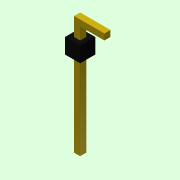
# Autodesk Inventor part: Pin-connector-angled
Saved by Autodesk Inventor 2015 (Build 190159000, 159)
## iProperties
Created: 2015-06-24
Part Number: Pin-connector-angled
Material: Generic
Document SubType Name: Modeling
Designer: Openlab
Density: 1 g/cm^3
Appearance: Default
Author: Openlab
Autodesk Inventor part; units mm, degrees
ref_plane "YZ Plane" through (0, 0, 0) normal (1, 0, 0) x (0, 1, 0)
ref_plane "XZ Plane" through (0, 0, 0) normal (0, 1, 0) x (-1, 0, 0)
ref_plane "XY Plane" through (0, 0, 0) normal (0, 0, 1) x (1, 0, 0)
sketch "Sketch1" plane through (0, 0, 0) normal (0, 1, 0) x (-1, 0, 0)
  line L0 (0, 0) -> (5, 0)
  line L1 (5, 0) -> (5, -19.5)
  line L2 (5, -19.5) -> (4, -19.5)
  line L3 (4, -19.5) -> (4, -1)
  line L4 (4, -1) -> (0, -1)
  line L5 (0, -1) -> (0, 0)
  line L6 (5.75, -3) -> (3.25, -3)
  line L7 (3.25, -3) -> (3.25, -5.5)
  line L8 (3.25, -5.5) -> (5.75, -5.5)
  line L9 (5.75, -5.5) -> (5.75, -3)
  line L10 (4.5, -1.8535) -> (4.5, -3.6396) construction
  dimension "d0" = 4
  dimension "d1" = 5
  dimension "d2" = 2.5
  dimension "d3" = 2.5
  dimension "d4" = 2
  dimension "d5" = 14
  dimension "d14" = 19.5
  constraints: 22 end point, 7 perpendicular, 1 horizontal, 1 vertical, 2 other
  measures "d0" distance between parallel lines of L5 L3
  measures "d1" distance between parallel lines of L5 L1
  measures "d2" distance of L8.end L6.start
  measures "d3" distance of L6.start L6.end
  measures "d4" distance between parallel lines of L6 L4
  measures "d5" distance between parallel lines of L2 L8
  measures "d14" distance between parallel lines of L2 L0
extrude "Extrusion1" add sketch "Sketch1" along normal blind 0.5 and the other way blind 0.5 contours L0 L1 L6 L3 L4 L5 | L1 L8 L3 L6 | L1 L2 L3 L8
extrude "Extrusion2" add sketch "Sketch1" against normal blind 1.25 and the other way blind 1.25 contours L6 L9 L8 L1 | L1 L8 L3 L6 | L3 L8 L7 L6
body "Solid1"
